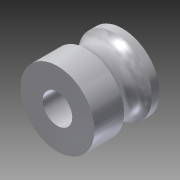
# Autodesk Inventor part: zebatka
Saved by Autodesk Inventor 2013 (Build 170138000, 138)
## iProperties
Created: 2014-04-23
Part Number: zebatka
Material: Generic
Document SubType Name: Modeling
Designer: Masta
Density: 1 g/cm^3
Author: Masta
Autodesk Inventor part; units mm, degrees
ref_plane "YZ Plane" through (0, 0, 0) normal (1, 0, 0) x (0, 1, 0)
ref_plane "XZ Plane" through (0, 0, 0) normal (0, 1, 0) x (-1, 0, 0)
ref_plane "XY Plane" through (0, 0, 0) normal (0, 0, 1) x (1, 0, 0)
sketch "Sketch1" plane through (0, 0, 0) normal (0, 0, 1) x (1, 0, 0)
  line L0 (0, 0) -> (0, 11)
  line L1 (0, 11) -> (6.25, 11)
  line L2 (6.25, 11) -> (6.25, 9.7)
  line L3 (0, 0) -> (6.25, 0)
  line L4 (6.25, 0) -> (6.25, 5)
  arc A0 (6.25, 9.7) -> (6.25, 5) centre (8.5112, 7.35) ccw
  line L5 (2.5, 0) -> (2.5, 11)
  dimension "d0" = 11
  dimension "d1" = 6.25
  dimension "d2" = 1.3
  dimension "d3" = 5
  dimension "d4" = 5.25
  dimension "d5" = 2.5
  constraints: 12 end point, 5 perpendicular, 2 point on circle, 2 point on line, 1 centre point, 1 collinear, 1 vertical
  measures "d0" distance of L0.start L0.end
  measures "d1" distance of L0.end L1.end
  measures "d2" distance of L1.end L2.end
  measures "d3" distance of L3.end L4.end
  measures "d4" distance edge to line of A0 L0
  measures "d5" distance between parallel lines of L0 L5
revolve "Revolution1" add sketch "Sketch1" angle 360 about axis through (0, 0, 0) along (0, 1, 0) contours L5 L1 L2 A0 L4 L3
body "Solid1"
